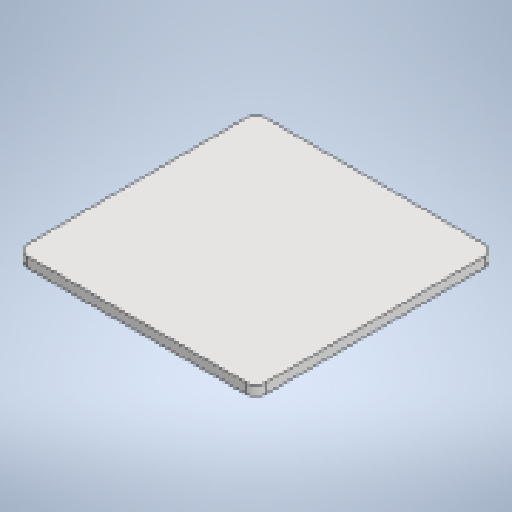
# Autodesk Inventor part: TKS 3532 FDS way cup
Saved by Autodesk Inventor 2025 (Build 290162010, 162A)
## iProperties
Created: 2025-06-24
Part Number: TKS 3532 FDS way cup
Material: Stainless Steel
Document SubType Name: Sheet Metal
Designer: user
Mass: 14.3451 g
Surface Area: 20.2627 cm^2
Volume: 1.79313 cm^3
Density: 8 g/cm^3
Flat Pattern Width: 4.8 cm
Flat Pattern Length: 4.8 cm
Flat Pattern Area: 23.04 cm^2
Sheet Metal Rule: AISI304 2mm Die16
Sheet Metal Width: 48,000 mm
Sheet Metal Length: 48,000 mm
Sheet Metal Area: 2304,000 mm^2
Appearance: Default
Author: user
Autodesk Inventor part; units mm, degrees
ref_plane "YZ Plane" through (0, 0, 0) normal (1, 0, 0) x (0, 1, 0)
ref_plane "XZ Plane" through (0, 0, 0) normal (0, 1, 0) x (-1, 0, 0)
ref_plane "XY Plane" through (0, 0, 0) normal (0, 0, 1) x (1, 0, 0)
sketch "Sketch1" plane through (0, 0, 0) normal (0, 0, 1) x (1, 0, 0)
  line L0 (-24, -24) -> (24, -24)
  line L1 (24, -24) -> (24, 24)
  line L2 (24, 24) -> (-24, 24)
  line L3 (-24, 24) -> (-24, -24)
  line L4 (-24, -24) -> (24, 24) construction
  line L5 (24, -24) -> (-24, 24) construction
  point P0 (0, 0)
  dimension "d154" = 48
  dimension "d155" = 48
  measures "d154" distance of L1.end L2.end
  measures "d155" distance of L0.end L1.end
extrude "Plate5" add sketch "Sketch1" along normal blind 2
fillet "Corner Round1" radius 2 4 edges at (24, 24, 1) (-24, 24, 1) (-24, -24, 1) (24, -24, 1)
body "Solid3"
